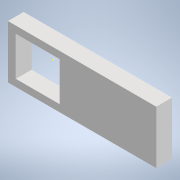
# Autodesk Inventor part: Pieza3
Saved by Autodesk Inventor 2020 (Build 240168000, 168)
## iProperties
Created: 2021-01-20
Part Number: Pieza3
Material: Genérico
Document SubType Name: Modeling
Designer: DanielAlvaradoPelaez
Density: 1 g/cm^3
Appearance: Valor por defecto
Author: DanielAlvaradoPelaez
Autodesk Inventor part; units mm, degrees
ref_plane "YZ Plane" through (0, 0, 0) normal (1, 0, 0) x (0, 1, 0)
ref_plane "XZ Plane" through (0, 0, 0) normal (0, 1, 0) x (-1, 0, 0)
ref_plane "XY Plane" through (0, 0, 0) normal (0, 0, 1) x (1, 0, 0)
sketch "Boceto1" plane through (0, 0, 0) normal (0, 0, 1) x (1, 0, 0)
  point P0 (0, 0)
sketch "Boceto2" plane through (0, 0, 0) normal (0, 0, 1) x (1, 0, 0)
  line L0 (-7.0268, -6.2798) -> (7.0268, -6.2798)
  line L1 (7.0268, -6.2798) -> (7.0268, 6.2798)
  line L2 (7.0268, 6.2798) -> (-7.0268, 6.2798)
  line L3 (-7.0268, 6.2798) -> (-7.0268, -6.2798)
  line L4 (-7.0268, -6.2798) -> (7.0268, 6.2798) construction
  line L5 (7.0268, -6.2798) -> (-7.0268, 6.2798) construction
  line L6 (-9.5542, -8.5385) -> (-9.5542, 8.5385)
  line L7 (-9.5542, 8.5385) -> (38.1222, 8.5385)
  line L8 (38.1222, 8.5385) -> (38.1222, -8.5385)
  line L9 (38.1222, -8.5385) -> (-9.5542, -8.5385)
  point P0 (0, 0)
  constraints: 20 end point, 4 parallel, 2 midpoint, 2 perpendicular, 1 horizontal, 1 vertical
extrude "Extrusión1" add sketch "Boceto2" along normal blind 5.08
